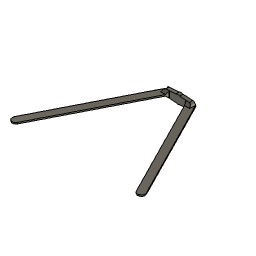
tail prototype assembly (Autodesk Fusion 360 archive; units mm, degrees)
design "tail"
Autodesk Fusion 360 part; units mm, degrees
sketch "Sketch1" plane through (0, 0, 0) normal (0, 1, 0) x (1, 0, 0)
  line L0 (1.8028, -3) -> (13.8929, -2.2456)
  line L1 (1.8028, 3) -> (13.8929, 2.2456)
  line L2 (-1.8028, -3) -> (-13.8929, -2.2456)
  line L3 (-1.8028, 3) -> (-13.8929, 2.2456)
  arc A0 (1.8028, 3) -> (-1.8028, 3) centre (0, 0) ccw
  arc A1 (-1.8028, -3) -> (1.8028, -3) centre (0, 0) ccw
  arc A2 (-13.8929, 2.2456) -> (-13.8929, -2.2456) centre (-13.7528, 0) ccw
  arc A3 (13.8929, -2.2456) -> (13.8929, 2.2456) centre (13.7528, 0) ccw
  arc A4 (-13.9863, 3.7427) -> (-13.9863, -3.7427) centre (-13.7528, 0) ccw
  line L4 (-2.2275, -4.4764) -> (-13.9863, -3.7427)
  arc A5 (-2.2275, -4.4764) -> (2.2275, -4.4764) centre (0, 0) ccw
  line L5 (2.2275, -4.4764) -> (13.9863, -3.7427)
  arc A6 (13.9863, -3.7427) -> (13.9863, 3.7427) centre (13.7528, 0) ccw
  line L6 (2.2275, 4.4764) -> (13.9863, 3.7427)
  arc A7 (2.2275, 4.4764) -> (-2.2275, 4.4764) centre (0, 0) ccw
  line L7 (-2.2275, 4.4764) -> (-13.9863, 3.7427)
  dimension "d1" = 7
  dimension "d3" = 4.5
  dimension "d4" = -1.5
  constraint coincident A0.centre A1.centre
  constraint tangent L0 A3
  constraint tangent L1 A3
  constraint concentric A0 A1
  measures "d1" diameter of A0
  measures "d3" diameter of A3
extrude "Extrude1" add sketch "Sketch1" along normal blind 2.5
extrude "Extrude2" add sketch "Sketch1" against normal blind 1.5 contours L0 L1 L2 L3 A0 A1 A2 A3 | A4 L4 A5 L5 A6 L6 A7 L7
sketch "Sketch2" plane through (0, 0, 0) normal (0, 0, 1) x (1, 0, 0)
  line L0 (-22.0607, -6.021) -> (-78.9733, -117.9802)
  arc A0 (-78.9733, -117.9802) -> (-71.0267, -122.0198) centre (-75, -120) ccw
  line L1 (-71.0267, -122.0198) -> (-10.0267, -2.0198)
  line L2 (-14, 0) -> (-75, -120) construction
  line L3 (-17.5, 2.5) -> (-17.5, -1.5)
  line L4 (-17.5, -1.5) -> (-9, -1.5)
  arc A1 (-10.0267, -2.0198) -> (-9.8028, -1.5) centre (-14, 0) ccw
  line L5 (-17.5, 2.5) -> (-22.0607, -6.021)
  line L6 (22.0607, -6.021) -> (78.9733, -117.9802)
  line L7 (71.0267, -122.0198) -> (10.0267, -2.0198)
  arc A2 (71.0267, -122.0198) -> (78.9733, -117.9802) centre (75, -120) ccw
  line L8 (17.5, 2.5) -> (22.0607, -6.021)
  line L9 (17.5, 2.5) -> (17.5, -1.5)
  line L10 (17.5, -1.5) -> (9, -1.5)
  arc A3 (9.8028, -1.5) -> (10.0267, -2.0198) centre (14, 0) ccw
  dimension "d9" = 14
  constraint tangent L0 A0
  constraint tangent A0 L1
  constraint parallel L0 L1
  constraint tangent L1 A1
  constraint tangent L0 A1
  constraint perpendicular L3 L4
  constraint coincident L4 A1.end
  measures "d9" distance of origin L2.start
extrude "Extrude3" add sketch "Sketch2" along normal mid plane 1.5
chamfer "Chamfer1" distance 3.2 angle 45 4 edges at (-13.6149, -1.5, 0.75) (-13.6149, -1.5, -0.75) (13.6149, -1.5, -0.75) (13.6149, -1.5, 0.75)

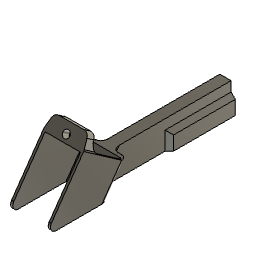
design "servo case"
Autodesk Fusion 360 part; units mm, degrees
ref_plane "WorkPlane1" through (12.125, 0, 0) normal (0, -0.819152, 0.573576) x (1, 0, 0)
sketch "Sketch1" plane through (0, 0, 0) normal (0, -0.819152, 0.573576) x (1, 0, 0)
  circle A0 centre (0, 13.75) radius 1.25
  line L0 (-6, 17) -> (6, 17)
  line L1 (6.3, -11.25) -> (6.3, 11.55)
  line L2 (6.3, 11.55) -> (-6.3, 11.55)
  line L3 (-6.3, 11.55) -> (-6.3, -11.25)
  line L4 (7.1, -11.25) -> (7.1, 12.35)
  line L5 (-7.1, 12.35) -> (-7.1, -11.25)
  line L6 (-6, 17) -> (-7.1, 12.35)
  line L7 (6, 17) -> (7.1, 12.35)
  line L8 (-7.1, -11.25) -> (-6.3, -11.25)
  line L9 (6.3, -11.25) -> (7.1, -11.25)
  line L10 (-6.3, 11.55) -> (6.3, 11.55)
  line L11 (6.3, 11.55) -> (6.3, -11.25)
  line L12 (6.3, -11.25) -> (-6.3, -11.25)
  line L13 (-6.3, -11.25) -> (-6.3, 11.55)
  dimension "d5" = 2.5
  constraint horizontal L0
  constraint perpendicular L1 L8
  constraint coincident L4.start L8
  constraint collinear L8 L9
  constraint horizontal L10
  constraint vertical L11
  constraint horizontal L12
  constraint vertical L13
  measures "d5" diameter of A0
extrude "Extrude1" add sketch "Sketch1" against normal blind 10 contours L0 L1 L2 L3 L4 L5 L6 L7 L8 L9 L10 L11 L13 picked at (-4.512013, 14.162101)
sketch "Sketch2" plane through (0, 0, 0) normal (1, 0, 0) x (0, 1, 0)
  line L0 (8, 0) -> (8, 5)
  line L1 (8, 5) -> (58, 5)
  line L2 (58, 5) -> (58, -2)
  line L3 (38, -5) -> (8, -5)
  line L4 (8, -5) -> (8, 5)
  line L5 (38, -5) -> (38, -2)
  line L6 (38, -2) -> (58, -2)
  dimension "d11" = 5
  dimension "d12" = 50
  constraint horizontal L1
  constraint vertical L2
  constraint horizontal L3
  constraint vertical L4
  constraint vertical L5
  constraint horizontal L6
  measures "d11" distance of L0.start L0.end
  measures "d12" distance of L0.end L1.end
extrude "Extrude2" add 1 faces at (-4.512013, 8.123047, 11.600914) along direction (0, -0.81915204, 0.57357644) blind 8
sketch "Sketch3" plane through (-6.3, 0, 0) normal (1, 0, 0) x (0, 1, 0)
  line L0 (-13.005951, -4.626849) -> (1.738786, -14.951225)
  line L1 (1.738786, -14.951225) -> (14.816328, 3.725442)
  line L2 (14.816328, 3.725442) -> (0.071591, 14.049818)
  line L3 (0.071591, 14.049818) -> (-13.005951, -4.626849)
  line L4 (14.033052, 4.273898) -> (0.955509, -14.402769)
  constraint perpendicular L0 L4
extrude "Extrude3" add sketch "Sketch3" along normal blind 12.893 contours L0 L1 L2 L4 picked at (5.836874, -8.542851)
extrude "Extrude4" add sketch "Sketch2" along normal mid plane 4 contours L0 L1 L2 L3 L4 L5 L6 picked at (34.666667, 2.666667)
sketch "Sketch4" plane through (0, 0, 0) normal (1, 0, 0) x (0, 1, 0)
  line L0 (10, -5) -> (-15.477592, -5)
  line L1 (-15.477592, -5) -> (-15.477592, -10)
  line L2 (-15.477592, -10) -> (-15.477592, -20)
  line L3 (-15.477592, -20) -> (10, -20)
  line L4 (10, -20) -> (10, -5)
  constraint horizontal L0
  constraint perpendicular L0 L1
  constraint parallel L1 L2
  constraint perpendicular L2 L3
  constraint perpendicular L0 L4
extrude "Extrude5" cut sketch "Sketch4" along normal mid plane 400 contours L0 L1 L2 L3 L4 picked at (1.50747, -11.666667)
extrude "Extrude6" cut 1 faces at (6.3, -1.620682, 1.349939) along direction (-1, 0, 0) blind 9.148
fillet "Fillet1" radius 2 6 edges at (6, 10.569952, 13.352009) (-6, 10.569952, 13.352009) (7.1, 7.902821, 9.542951) (-7.1, 7.902821, 9.542951) (-2, 12.207746, 0) (2, 12.207746, 0)
fillet "Fillet2" radius 1.509 9 edges at (-7.1, 11.92403, -0.405188) (-7.086526, 15.274288, 4.379476) (-6.705244, 16.23234, 5.747717) (-5.658721, 17.694862, 7.836414) (0, 17.94232, 8.189821) (5.658721, 17.694862, 7.836414) (6.705244, 16.23234, 5.747717) (7.086526, 15.274288, 4.379476) (7.1, 11.92403, -0.405188)
fillet "Fillet3" radius 2 2 faces at (6.833333, -12.828313, -4.751233) (-6.833333, -12.828313, -4.751233)
sketch "Sketch5" plane through (2, 0, 0) normal (1, 0, 0) x (0, 1, 0)
  line L0 (18.150333, 5) -> (11.148257, -5)
  line L1 (11.148257, -5) -> (38, -5)
  line L2 (38, -5) -> (38, -2)
  line L3 (38, -2) -> (58, -2)
  line L4 (58, -2) -> (58, 5)
  line L5 (58, 5) -> (18.150333, 5)
  line L6 (36.000001, 0) -> (58.000001, 0)
  line L7 (58.000001, 0) -> (58.000001, -5)
  line L8 (58.000001, -5) -> (36.000001, -5)
  line L9 (36.000001, -5) -> (36.000001, 0)
  constraint horizontal L6
  constraint vertical L7
  constraint horizontal L8
  constraint vertical L9
extrude "Extrude7" add sketch "Sketch5" along normal blind 1.5 contours L1 L2 L3 L4 L6 L7 L8 L9 | L2 L3 L7 L8 picked at (44, -0.666667) picked at (51.333334, -4)
chamfer "Chamfer1" distance 1.5 angle 45 2 edges at (2, 47.000001, 0) (2, 36.000001, -2.5)
sketch "Sketch6" plane through (-2, 0, 0) normal (-1, 0, 0) x (0, -1, 0)
  line L0 (-11.148257, -5) -> (-18.150333, 5)
  line L1 (-18.150333, 5) -> (-58, 5)
  line L2 (-58, 5) -> (-58, -2)
  line L3 (-58, -2) -> (-38, -2)
  line L4 (-38, -2) -> (-38, -5)
  line L5 (-38, -5) -> (-11.148257, -5)
  line L6 (-36.000001, 0) -> (-58.000001, 0)
  line L7 (-58.000001, 0) -> (-58.000001, -5)
  line L8 (-58.000001, -5) -> (-36.000001, -5)
  line L9 (-36.000001, -5) -> (-36.000001, 0)
  constraint horizontal L6
  constraint vertical L7
  constraint horizontal L8
  constraint vertical L9
extrude "Extrude8" add sketch "Sketch6" along normal blind 1.5 contours L2 L3 L4 L5 L6 L7 L8 L9 | L3 L4 L7 L8 picked at (-44.000001, -0.666667) picked at (-51.333334, -4)
chamfer "Chamfer2" distance 1.5 angle 45 2 edges at (-2, 47.000001, 0) (-2, 36.000001, -2.5)
ref_plane "WorkPlane2" through (0, -1.475539, 6.609945) normal (0, -0.819152, 0.573576) x (1, 0, 0)
sketch "Sketch7" plane through (0, -4.09576, 2.867882) normal (0, -0.819152, 0.573576) x (1, 0, 0)
  line L0 (6.3, -9.59562) -> (7.1, -9.59562)
  line L1 (7.1, -9.59562) -> (7.1, 12.116661)
  arc A0 (7.1, 12.116661) -> (7.046284, 12.577072) centre (5.1, 12.116661) ccw
  line L2 (7.046284, 12.577072) -> (6.364204, 15.460411)
  arc A1 (6.364204, 15.460411) -> (4.41792, 17) centre (4.41792, 15) ccw
  line L3 (4.41792, 17) -> (-4.41792, 17)
  arc A2 (-4.41792, 17) -> (-6.364204, 15.460411) centre (-4.41792, 15) ccw
  line L4 (-6.364204, 15.460411) -> (-7.046284, 12.577072)
  arc A3 (-7.046284, 12.577072) -> (-7.1, 12.116661) centre (-5.1, 12.116661) ccw
  line L5 (-7.1, 12.116661) -> (-7.1, -9.59562)
  line L6 (-7.1, -9.59562) -> (-6.3, -9.59562)
  line L7 (-6.3, -9.59562) -> (-6.3, 11.55)
  line L8 (-6.3, 11.55) -> (6.3, 11.55)
  line L9 (6.3, 11.55) -> (6.3, -9.59562)
  circle A4 centre (0, 13.75) radius 1.25
  line L10 (-7.1, 12.116661) -> (7.1, 12.116661)
  constraint perpendicular L1 L10
extrude "Extrude9" cut sketch "Sketch7" against normal blind 12.979 contours A0 L2 A1 L3 A2 L4 A3 L10 picked at (-4.882175, 13.86706)
sketch "Sketch8" plane through (0, 6.624808, 9.461206) normal (0, -0.573576, -0.819152) x (1, 0, 0)
  line L0 (6.3, 8) -> (-6.3, 8)
  line L1 (-6.3, 8) -> (-6.3, -9.043796)
  line L2 (-6.3, -9.043796) -> (6.3, -9.043796)
  line L3 (6.3, -9.043796) -> (6.3, 8)
  line L4 (-6.3, 8) -> (6.3, 8)
  line L5 (6.3, 8) -> (6.3, 5)
  line L6 (6.3, 5) -> (-6.3, 5)
  line L7 (-6.3, 5) -> (-6.3, 8)
  dimension "d40" = 3
  constraint horizontal L4
  constraint vertical L5
  constraint horizontal L6
  constraint vertical L7
  constraint coincident L0.end L1.start
  measures "d40" distance of L0.end L6.end
extrude "Extrude10" cut sketch "Sketch8" against normal blind 10.881 contours L1 L2 L3 L6 picked at (2.1, -4.362531)
sketch "Sketch9" plane through (0, 0, 0) normal (1, 0, 0) x (0, 1, 0)
  line L0 (20, 5) -> (11.5, 5)
  line L1 (14, 5) -> (2.875771, 12.783158)
  line L2 (2.875771, 12.783158) -> (20, 10.5)
  line L3 (20, 10.5) -> (20, 5)
  constraint horizontal L0
  constraint coincident L0 L1.start
  constraint perpendicular L0 L3
extrude "Extrude11" cut sketch "Sketch9" along normal mid plane 60 contours L0 L1 L2 L3 picked at (12.291924, 9.427719)
fillet "Fillet4" radius 3.165 2 edges at (6.7, 2.854071, 12.79327) (-6.7, 2.854071, 12.79327)
